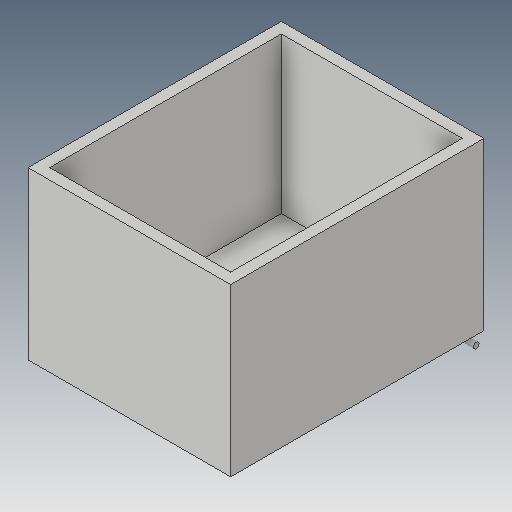
# Autodesk Inventor part: Body
Saved by Autodesk Inventor 2019 (Build 230136000, 136)
## iProperties
Created: 2019-04-28
Part Number: Body
Material: 일반
Document SubType Name: Modeling
Designer: hinmo
Density: 1 g/cm^3
Appearance: 기본값
Author: hinmo
Autodesk Inventor part; units mm, degrees
ref_plane "YZ Plane" through (0, 0, 0) normal (1, 0, 0) x (0, 1, 0)
ref_plane "XZ Plane" through (0, 0, 0) normal (0, 1, 0) x (-1, 0, 0)
ref_plane "XY Plane" through (0, 0, 0) normal (0, 0, 1) x (1, 0, 0)
sketch "스케치1" plane through (0, 0, 0) normal (1, 0, 0) x (0, 1, 0)
  line L0 (-230, 350) -> (230, 350)
  line L1 (230, 350) -> (230, -350)
  line L2 (230, -350) -> (-230, -350)
  line L3 (-230, -350) -> (-230, 350)
  line L4 (-230, 350) -> (230, -350) construction
  line L5 (230, 350) -> (-230, -350) construction
  circle A0 centre (-255, -328.5) radius 8
  point P0 (0, 0)
  dimension "d0" = 460
  dimension "d1" = 700
  dimension "d4" = 16
  dimension "d5" = 25
  dimension "d7" = 21.5
  constraints: 12 end point, 2 midpoint, 2 parallel, 1 centre point, 1 horizontal, 1 perpendicular
  measures "d0" distance of L1.end L2.end
  measures "d1" distance of L0.end L1.end
  measures "d4" diameter of A0
  measures "d5" distance from line of L3 A0.centre
  measures "d7" distance from line of L2 A0.centre
extrude "돌출2" add sketch "스케치1" along normal blind 560
sketch "스케치2" plane through (0, 230, 350) normal (0, 1, 0) x (1, 0, 0)
  line L0 (0, 700) -> (0, 0) projected
  line L1 (560, 0) -> (560, 700) projected
  line L2 (0, 0) -> (560, 700)
  line L3 (560, 0) -> (0, 700)
  line L4 (530, 30) -> (30, 30)
  line L5 (30, 30) -> (30, 670)
  line L6 (30, 670) -> (530, 670)
  line L7 (530, 670) -> (530, 30)
  line L8 (530, 30) -> (30, 670) construction
  line L9 (30, 30) -> (530, 670) construction
  point P0 (0, 350)
  point P1 (280, 350)
  dimension "d10" = 500
  dimension "d11" = 640
  constraints: 16 end point, 3 midpoint, 2 parallel, 1 horizontal, 1 perpendicular
  measures "d10" distance of L5.end L6.end
  measures "d11" distance of L4.end L5.end
extrude "돌출3" cut sketch "스케치2" against normal blind 430 contours L5 L6 L7 L2 L3 | L3 L2 L5 | L2 L3 L7 L4 L5 | L2 L7 L3
